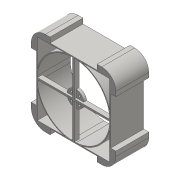
# Autodesk Inventor part: Motor mount (plain)
Saved by Autodesk Inventor 2016 (Build 200138000, 138)
## iProperties
Created: 2016-03-10
Part Number: Motor mount (plain)
Material: Generic
Document SubType Name: Modeling
Designer: s_sud
Density: 1 g/cm^3
Appearance: Default
Author: s_sud
Autodesk Inventor part; units mm, degrees
ref_plane "YZ Plane" through (0, 0, 0) normal (1, 0, 0) x (0, 1, 0)
ref_plane "XZ Plane" through (0, 0, 0) normal (0, 1, 0) x (-1, 0, 0)
ref_plane "XY Plane" through (0, 0, 0) normal (0, 0, 1) x (1, 0, 0)
sketch "Sketch1" plane through (0, 0, 0) normal (0, 1, 0) x (-1, 0, 0)
  circle A0 centre (0, 0) radius 38.5
  circle A1 centre (0, 0) radius 39.5
  dimension "d0" = 77
  dimension "d1" = 79
  constraints: 2 centre point, 2 coincident
  measures "d0" diameter of A0
  measures "d1" diameter of A1
extrude "Extrusion1" add sketch "Sketch1" along normal blind 35
sketch "Sketch12" plane through (0, 0, 0) normal (0, -1, 0) x (1, 0, 0)
  line L0 (-1, -39) -> (1, -39)
  line L1 (1, -39) -> (1, 39)
  line L2 (1, 39) -> (-1, 39)
  line L3 (-1, 39) -> (-1, -39)
  line L4 (-1, -39) -> (1, 39) construction
  line L5 (1, -39) -> (-1, 39) construction
  line L6 (-39, -1) -> (39, -1)
  line L7 (39, -1) -> (39, 1)
  line L8 (39, 1) -> (-39, 1)
  line L9 (-39, 1) -> (-39, -1)
  line L10 (-39, -1) -> (39, 1) construction
  line L11 (39, -1) -> (-39, 1) construction
  point P0 (0, 0)
  dimension "d64" = 78
  dimension "d65" = 2
  dimension "d66" = 78
  dimension "d67" = 2
  constraints: 24 end point, 4 midpoint, 4 parallel, 2 horizontal, 2 perpendicular
  measures "d64" distance of L0.end L1.end
  measures "d65" distance of L0.start L0.end
  measures "d66" distance of L7.end L8.end
  measures "d67" distance of L6.end L7.end
extrude "Extrusion12" add sketch "Sketch12" against normal blind 5
sketch "Sketch13" plane through (0, 5, 0) normal (0, 1, 0) x (1, 0, 0)
  circle A0 centre (0, 0) radius 9
  circle A1 centre (0, 6) radius 1
  circle A2 centre (-4.2426, 4.2426) radius 1
  circle A3 centre (-6, 0) radius 1
  circle A4 centre (-4.2426, -4.2426) radius 1
  circle A5 centre (0, -6) radius 1
  circle A6 centre (4.2426, -4.2426) radius 1
  circle A7 centre (6, 0) radius 1
  circle A8 centre (4.2426, 4.2426) radius 1
  dimension "d70" = 18
  dimension "d71" = 2
  dimension "d72" = 6
  dimension "d75" = 360
  constraints: 9 centre point, 1 coincident, 17 other
  measures "d70" diameter of A0
  measures "d71" diameter of A1
  measures "d72" distance of point (0, 0) A1.centre
extrude "Extrusion13" add sketch "Sketch13" against normal blind 3 contours A0 | A1 | A3 | A5 | A7
sketch "Sketch24" plane through (0, 35, 0) normal (0, 1, 0) x (1, 0, 0)
  line L0 (-39.5, -39.5) -> (39.5, -39.5)
  line L1 (39.5, -39.5) -> (39.5, 39.5)
  line L2 (39.5, 39.5) -> (-39.5, 39.5)
  line L3 (-39.5, 39.5) -> (-39.5, -39.5)
  line L4 (30, -45) -> (-30, -45)
  line L5 (-45, -30) -> (-45, 30)
  line L6 (-30, 45) -> (30, 45)
  line L7 (45, 30) -> (45, -30)
  line L8 (45, -45) -> (-45, 45) construction
  line L9 (-45, -45) -> (45, 45) construction
  arc A0 (-30, 45) -> (-45, 30) centre (-30, 30) ccw
  arc A1 (45, 30) -> (30, 45) centre (30, 30) ccw
  arc A2 (30, -45) -> (45, -30) centre (30, -30) ccw
  arc A3 (-45, -30) -> (-30, -45) centre (-30, -30) ccw
  line L10 (-25, -45) -> (-25, -39.5)
  line L11 (25, -45) -> (25, -39.5)
  line L12 (-45, -25) -> (-39.5, -25)
  line L13 (-45, 25) -> (-39.5, 25)
  line L14 (-25, 39.5) -> (-25, 45)
  line L15 (25, 39.5) -> (25, 45)
  line L16 (39.5, -25) -> (45, -25)
  line L17 (39.5, 25) -> (45, 25)
  line L18 (38.4008, -38.4008) -> (-38.4008, -38.4008)
  line L19 (-38.4008, -38.4008) -> (-38.4008, 38.4008)
  line L20 (-38.4008, 38.4008) -> (38.4008, 38.4008)
  line L21 (38.4008, 38.4008) -> (38.4008, -38.4008)
  line L22 (38.4008, -38.4008) -> (-38.4008, 38.4008) construction
  line L23 (-38.4008, -38.4008) -> (38.4008, 38.4008) construction
  line L24 (0, -45) -> (0, -39.5)
  line L25 (-45, 0) -> (-39.5, 0)
  line L26 (0, -38.4008) -> (0, 38.4008)
  line L27 (0, 39.5) -> (0, 45)
  line L28 (-38.4008, 0) -> (38.4008, 0)
  line L29 (39.5, 0) -> (45, 0)
  point P0 (0, 0)
  dimension "d133" = 79
  dimension "d134" = 79
  dimension "d135" = 90
  dimension "d136" = 90
  dimension "d137" = 15
  dimension "d149" = 25
  dimension "d150" = 25
  dimension "d151" = 38.4008
  dimension "d152" = 39.5
  dimension "d153" = 25
  dimension "d154" = 5.5
  dimension "d155" = 25
  dimension "d156" = 25
  dimension "d157" = 25
  dimension "d158" = 25
  dimension "d159" = 25
  constraints: 60 end point, 25 point on line, 16 midpoint, 11 perpendicular, 8 point on circle, 8 tangent, 6 parallel, 4 centre point, 3 equal radius, 3 horizontal
  measures "d133" distance of L2.end L0.start
  measures "d134" distance of L1.end L2.end
  measures "d135" distance of L9.start L8.end
  measures "d136" distance of L8.start L9.start
  measures "d137" radius of A0
  measures "d149" distance between parallel lines of L25 L13
  measures "d150" distance between parallel lines of L12 L25
  measures "d151" distance between parallel lines of L28 L20
  measures "d152" distance between parallel lines of L28 L2
  measures "d153" distance between parallel lines of L29 L17
  measures "d154" distance of L29.start L29.end
  measures "d155" distance between parallel lines of L16 L29
  measures "d156" distance between parallel lines of L24 L10
  measures "d157" distance between parallel lines of L24 L11
  measures "d158" distance between parallel lines of L27 L14
  measures "d159" distance between parallel lines of L27 L15
extrude "Extrusion24" add sketch "Sketch24" against normal blind 35 contours L3 L2 L1 L0 | L0 L10 L4 A3 L5 L12 L3 | L0 L1 L16 L7 A2 L4 L11 | L13 L5 A0 L6 L14 L2 L3 | L1 L2 L15 L6 A1 L7 L17
body "Solid1"
